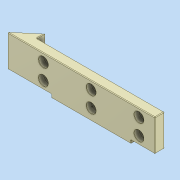
# Autodesk Inventor part: Platt unten
Saved by Autodesk Inventor 2021 (Build 250183000, 183)
## iProperties
Created: 2024-03-13
Part Number: Platt unten
Material: Generic
Document SubType Name: Modeling
Designer: Nokia
Density: 1 g/cm^3
Appearance: Smooth - Ash
Mass: 10895.6 g
Surface Area: 5905.84 cm^2
Volume: 10895.6 cm^3
Author: Nokia
Autodesk Inventor part; units mm, degrees
ref_plane "YZ Plane" through (0, 0, 0) normal (1, 0, 0) x (0, 1, 0)
ref_plane "XZ Plane" through (0, 0, 0) normal (0, 1, 0) x (-1, 0, 0)
ref_plane "XY Plane" through (0, 0, 0) normal (0, 0, 1) x (1, 0, 0)
sketch "Sketch1" plane through (0, 0, 0) normal (0, 0, 1) x (1, 0, 0)
  line L0 (-400, -120) -> (-400, 100)
  line L1 (-400, 100) -> (400, 100)
  line L2 (400, 100) -> (400, -120)
  line L3 (400, -120) -> (-400, -120)
  line L4 (0, 0) -> (0, 50)
  circle A0 centre (0, 50) radius 20
  line L5 (0, 0) -> (-150, 0)
  line L6 (-150, 0) -> (-150, 100)
  line L7 (-400, 100) -> (400, 100)
  circle A1 centre (0, -50) radius 20
  circle A2 centre (-300, 50) radius 20
  circle A3 centre (-300, -50) radius 20
  circle A4 centre (300, 50) radius 20
  circle A5 centre (300, -50) radius 20
  line L8 (0, 0) -> (0, 50)
  circle A6 centre (0, 50) radius 17
  line L9 (0, 0) -> (-150, 0)
  line L10 (-150, 0) -> (-150, 100)
  line L11 (-400, 100) -> (400, 100)
  circle A7 centre (0, -50) radius 17
  circle A8 centre (-300, 50) radius 17
  circle A9 centre (-300, -50) radius 17
  circle A10 centre (300, 50) radius 17
  circle A11 centre (300, -50) radius 17
  circle A12 centre (0, 50) radius 20
  circle A13 centre (0, -50) radius 20
  circle A14 centre (-300, -50) radius 20
  circle A15 centre (-300, 50) radius 20
  circle A16 centre (300, 50) radius 20
  circle A17 centre (300, -50) radius 20
  dimension "d0" = 800
  dimension "d8" = 220
  dimension "d31" = 50
  dimension "d32" = 40
  dimension "d33" = 150
  dimension "d53" = 50
  dimension "d54" = 34
  dimension "d55" = 150
  dimension "d56" = 40
  constraints: 24 end point, 18 centre point, 15 symmetric about line, 4 perpendicular, 3 coincident, 3 vertical, 2 horizontal, 2 point on line, 15 other
  measures "d0" distance of L0.end L1.end
  measures "d8" distance of L1.end L2.end
  measures "d31" distance of L4.start L4.end
  measures "d32" diameter of A0
  measures "d33" distance of L4.start L5.end
  measures "d53" distance of L8.start L8.end
  measures "d54" diameter of A6
  measures "d55" distance of L8.start L9.end
  measures "d56" diameter of A12
extrude "Extrusion1" add sketch "Sketch1" along normal blind 60 contours L0 L1 L2 L3 | A0 | A1 | A2 | A3 | A4 | A5 | A6 | A7 | A8 | A9 | A10 | A11
sketch "Sketch2" plane through (-400, 100, 0) normal (0, 1, 0) x (1, 0, 0)
  line L0 (800, -60) -> (0, -60) projected
  line L1 (0, -60) -> (-131.0929, -60)
  line L2 (800, 0) -> (0, 0) projected
  line L3 (0, -60) -> (0, 50)
  line L4 (0, 0) -> (0, -60) projected
  line L5 (0, 50) -> (-131.0929, -60)
  point P0 (400, 0)
  dimension "d5" = 110
  dimension "d70" = 40
  constraints: 6 end point, 1 collinear, 1 horizontal
  measures "d5" distance of L0.end L3.end
  measures "d70" angle of L1 L5
extrude "Extrusion2" add sketch "Sketch2" against normal blind 200
sketch "Sketch4" plane through (0, 0, 0) normal (0, 0, -1) x (-1, 0, 0)
  line L0 (-50, -115) -> (-50, -105)
  line L1 (-50, -105) -> (50, -105)
  line L2 (50, -105) -> (50, -115)
  line L3 (50, -115) -> (-50, -115)
  line L4 (400, -120) -> (-400, -120) projected
  point P0 (0, 0)
  dimension "d17" = 100
  dimension "d20" = 10
  dimension "d21" = 15
  constraints: 8 end point, 2 perpendicular, 1 vertical, 1 other
  measures "d17" distance of L0.end L1.end
  measures "d20" distance of L0.start L0.end
extrude "Extrusion4" cut sketch "Sketch4" against normal blind 40
sketch "Sketch5" plane through (400, -120, 0) normal (0, -1, 0) x (1, 0, 0)
  line L0 (-400, 0) -> (-400, 40)
  line L1 (-350, 40) -> (-450, 40) projected
  line L2 (-400, 20) -> (-450, 20)
  line L3 (-450, 0) -> (-450, 40) projected
  line L4 (-800, 0) -> (0, 0) projected
  line L5 (-425, 0) -> (-425, 20)
  circle A0 centre (-425, 10) radius 5
  circle A1 centre (-425, 30) radius 5
  circle A2 centre (-375, 10) radius 5
  circle A3 centre (-375, 30) radius 5
  dimension "d22" = 10
  constraints: 6 end point, 5 midpoint, 4 centre point, 3 symmetric about line, 1 perpendicular, 1 point on line, 3 other
  measures "d22" diameter of A0
hole "Hole1" at (-25, -120, 10) at (-25, -120, 30) at (25, -120, 10) at (25, -120, 30) direction (0, 1, 0) diameter 10 depth 15
sketch "Sketch6" plane through (400, -120, 0) normal (1, 0, 0) x (0, 0, -1)
  line L0 (0, 5) -> (0, 15) projected
  line L1 (0, 0) -> (0, 15)
  point P0 (0, 120)
  constraints: 2 end point, 1 vertical
ref_plane "Work Plane1" through (400, -105, 0) normal (0, -1, 0) x (1, 0, 0)
sketch "Sketch7" plane through (400, -105, 0) normal (0, -1, 0) x (1, 0, 0)
  line L0 (-400, 0) -> (-400, 40)
  line L1 (-350, 40) -> (-450, 40)
  line L2 (-400, 20) -> (-450, 20)
  line L3 (-450, 0) -> (-450, 40)
  line L4 (-425, 0) -> (-425, 20)
  circle A0 centre (-425, 10) radius 5
  circle A1 centre (-425, 30) radius 5
  circle A2 centre (-375, 10) radius 5
  circle A3 centre (-375, 30) radius 5
  dimension "d30" = 10
  constraints: 10 end point, 5 midpoint, 4 centre point, 3 symmetric about line, 1 perpendicular, 3 other
  measures "d30" diameter of A0
extrude "Extrusion5" cut sketch "Sketch1" along normal blind 2 contours A0 | A1 | A2 | A3 | A4 | A5
extrude "Extrusion6" cut sketch "Sketch1" along normal through all contours A6 | A7 | A8 | A9 | A10 | A11
sketch "Sketch8" plane through (0, 0, 60) normal (0, 0, 1) x (1, 0, 0)
  line L0 (0, 0) -> (0, 50)
  line L1 (0, 0) -> (-150, 0)
  line L2 (-150, 0) -> (-150, 100)
  line L3 (-400, 100) -> (400, 100)
  circle A0 centre (0, 50) radius 30
  circle A1 centre (0, -50) radius 30
  circle A2 centre (-300, -50) radius 30
  circle A3 centre (-300, 50) radius 30
  circle A4 centre (300, 50) radius 30
  circle A5 centre (300, -50) radius 30
  dimension "d61" = 50
  dimension "d63" = 150
  dimension "d64" = 60
  constraints: 8 end point, 6 centre point, 5 symmetric about line, 1 horizontal, 1 perpendicular, 1 point on line, 1 vertical, 5 other
  measures "d61" distance of L0.start L0.end
  measures "d63" distance of L0.start L1.end
  measures "d64" diameter of A0
extrude "Extrusion7" cut sketch "Sketch8" against normal blind 32
sketch "Sketch9" plane through (-400, -120, 0) normal (0, -1, 0) x (1, 0, 0)
  line L0 (0, 0) -> (0, -50) projected
  line L1 (0, 0) -> (150, 0)
  line L2 (800, 0) -> (0, 0) projected
  line L3 (150, 0) -> (150, 60)
  line L4 (800, 60) -> (-131.0929, 60) projected
  line L5 (150, 60) -> (0, 60)
  line L6 (0, 60) -> (0, 0) projected
  line L7 (0, 60) -> (0, 0)
  line L8 (400, 0) -> (400, 60)
  line L9 (370, 60) -> (430, 60) projected
  line L10 (800, 0) -> (800, -50)
  line L11 (800, 0) -> (650, 0)
  line L12 (650, 0) -> (650, 60)
  line L13 (650, 60) -> (800, 60)
  line L14 (800, 60) -> (800, 0)
  line L15 (800, 60) -> (800, 0)
  dimension "d67" = 150
  constraints: 22 end point, 3 point on line, 3 symmetric about line, 1 collinear, 1 midpoint, 1 perpendicular
  measures "d67" distance of L0.start L1.end
extrude "Extrusion8" cut sketch "Sketch9" against normal blind 20 contours L6 L4 L3 L1 | L12 L4 L14 L2
hole "Hole3" at (-25, -105, 10) at (25, -105, 10) at (25, -105, 30) at (-25, -105, 30) direction (0, 1, 0) diameter 6.647 depth 38 tip angle 118 thread size "M8x1.25" class "6H" standard "ISO Metric profile"
fillet "Fillet2" radius 4 26 edges at (-400, -100, -25) (-400, 100, -25) (-465.5464, 100, 5) (-465.5464, -100, 5) (-531.0929, 0, 60) (-65.5464, 100, 60) (0, 100, 0) (400, 100, 30) (400, 0, 60) (400, 0, 0) (400, -100, 30) (325, -100, 60) (325, -100, 0) (250, -110, 0) (250, -110, 60) (250, -120, 30) (0, -120, 0) (0, -120, 60) (-250, -120, 30) (-250, -110, 0) (-250, -110, 60) (-390.5464, -100, 60) (-250, -100, 30) (250, -100, 30) (-325, -100, 0) (-400, 0, 0)
chamfer "Chamfer1" distance 2 angle 45 6 edges at (-330, 50, 60) (-330, -50, 60) (-30, 50, 60) (-30, -50, 60) (270, 50, 60) (270, -50, 60)
chamfer "Chamfer2" distance 0.5 angle 45 12 edges at (-320, 50, 0) (-317, 50, 2) (-320, -50, 0) (-317, -50, 2) (-20, -50, 0) (-17, -50, 2) (-20, 50, 0) (-17, 50, 2) (280, 50, 0) (283, 50, 2) (280, -50, 0) (283, -50, 2)
fillet "Fillet3" radius 4 8 edges at (0, -115, 40) (0, -105, 40) (-50, -110, 40) (-50, -115, 20) (-50, -105, 20) (50, -105, 20) (50, -110, 40) (50, -115, 20)
chamfer "Chamfer3" distance 1 angle 45 8 edges at (0, -105, 0) (-48.8284, -106.1716, 0) (-50, -110, 0) (-48.8284, -113.8284, 0) (0, -115, 0) (48.8284, -113.8284, 0) (50, -110, 0) (48.8284, -106.1716, 0)
chamfer "Chamfer4" distance 0.5 angle 45 4 edges at (25, -105, 13.3235) (25, -105, 33.3235) (-25, -105, 13.3235) (-25, -105, 33.3235)
body "Solid1"
